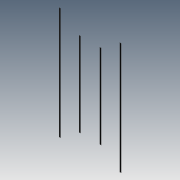
# Autodesk Inventor part: GE-12017-03
Saved by Autodesk Inventor 2012 (Build 160160000, 160)
## iProperties
Created: 2011-11-19
Part Number: GE-12017-03
Document SubType Name: Modeling
Designer: dfoster
Density: 1 g/cm^3
Material: Default
Author: dfoster
Autodesk Inventor part; units mm, degrees
ref_plane "YZ Plane" through (0, 0, 0) normal (1, 0, 0) x (0, 1, 0)
ref_plane "XZ Plane" through (0, 0, 0) normal (0, 1, 0) x (-1, 0, 0)
ref_plane "XY Plane" through (0, 0, 0) normal (0, 0, 1) x (1, 0, 0)
sketch "Sketch1" plane through (0, 0, 0) normal (0, 0, 1) x (1, 0, 0)
  line L0 (0, 0) -> (25.4, 0)
  line L1 (25.4, 0) -> (25.4, -2133.6)
  line L2 (25.4, -2133.6) -> (0, -2133.6)
  line L3 (0, -2133.6) -> (0, 0)
  line L4 (381, -266.7) -> (406.4, -266.7)
  line L5 (406.4, -266.7) -> (406.4, -1866.9)
  line L6 (406.4, -1866.9) -> (381, -1866.9)
  line L7 (381, -1866.9) -> (381, -266.7)
  line L8 (774.7, -266.7) -> (800.1, -266.7)
  line L9 (800.1, -266.7) -> (800.1, -1866.9)
  line L10 (800.1, -1866.9) -> (774.7, -1866.9)
  line L11 (774.7, -1866.9) -> (774.7, -266.7)
  line L12 (1155.7, 0) -> (1181.1, 0)
  line L13 (1181.1, 0) -> (1181.1, -2133.6)
  line L14 (1181.1, -2133.6) -> (1155.7, -2133.6)
  line L15 (1155.7, -2133.6) -> (1155.7, 0)
  dimension "d0" = 355.6
  dimension "d1" = 2133.6
  dimension "d2" = 1600.2
  dimension "d3" = 25.4
  dimension "d4" = 266.7
  dimension "d5" = 393.7
  dimension "d6" = 355.6
  constraints: 32 end point, 6 vertical, 4 collinear, 3 equal length, 3 horizontal
  measures "d0" distance between parallel lines of L7 L1
  measures "d1" distance of L2.end L0.start
  measures "d2" distance of L6.end L4.start
  measures "d3" distance between parallel lines of L1 L3
  measures "d4" distance between parallel lines of L0 L4
  measures "d5" distance between parallel lines of L11 L7
  measures "d6" distance between parallel lines of L9 L15
extrude "Extrusion1" add sketch "Sketch1" along normal blind 1.5875
equation "\"d4\" = -0.5 * d2 + 0.5 * d1"
body "Solid1"
